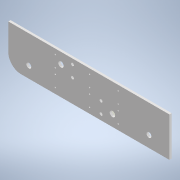
# Autodesk Inventor part: new sidewall inside
Saved by Autodesk Inventor 2020 (Build 240168000, 168)
## iProperties
Created: 2020-02-26
Part Number: new sidewall inside
Material: Generic
Document SubType Name: Modeling
Designer: jackm
Density: 1 g/cm^3
Appearance: Default
Author: jackm
Autodesk Inventor part; units mm, degrees
ref_plane "YZ Plane" through (0, 0, 0) normal (1, 0, 0) x (0, 1, 0)
ref_plane "XZ Plane" through (0, 0, 0) normal (0, 1, 0) x (-1, 0, 0)
ref_plane "XY Plane" through (0, 0, 0) normal (0, 0, 1) x (1, 0, 0)
ref_plane "Work Plane1" through (0, 0, 0) normal (0, 0, 1) x (1, 0, 0)
sketch "Sketch1" plane through (0, 0, 0) normal (0, 0, 1) x (1, 0, 0)
  circle A0 centre (104, 56) radius 1.778 construction
  circle A1 centre (104, 88) radius 1.778 construction
  circle A2 centre (184, 88) radius 1.778 construction
  line L0 (327.4055, 102.35) -> (327.4055, -7.6771) construction
  line L1 (-123.4445, 102.35) -> (327.4055, 102.35) construction
  line L2 (-123.4445, 27.6143) -> (-123.4445, 102.35) construction
  arc A3 (-123.4445, 27.6143) -> (-88.1531, -7.6771) centre (-88.1531, 27.6143) ccw construction
  line L3 (327.4055, -7.6771) -> (-88.1531, -7.6771) construction
  circle A4 centre (270.0149, 24.0729) radius 6.8857 construction
  circle A5 centre (-66.0538, 24.0729) radius 6.8834 construction
  circle A6 centre (168.0148, 24) radius 6.8834 construction
  circle A7 centre (23.9852, 72) radius 6.8834 construction
  line L4 (-123.4445, 102.35) -> (327.4055, 102.35)
  line L5 (327.4055, 102.35) -> (327.4055, -7.6771)
  line L6 (327.4055, -7.6771) -> (-88.1531, -7.6771)
  line L7 (-123.4445, 27.6143) -> (-123.4445, 102.35)
  arc A8 (-123.4445, 27.6143) -> (-88.1531, -7.6771) centre (-88.1531, 27.6143) ccw
  circle A9 centre (-66.0538, 24.0729) radius 6.8834
  circle A10 centre (270.0149, 24.0729) radius 6.8857
  circle A11 centre (23.9852, 72) radius 7.62
  circle A12 centre (168.0148, 24) radius 7.62
  circle A13 centre (56, 56) radius 3.5 construction
  circle A14 centre (136, 40) radius 3.5 construction
  circle A15 centre (136, 8) radius 3.5 construction
  circle A16 centre (56, 88) radius 3.5 construction
  circle A17 centre (56, 88) radius 4.064
  circle A18 centre (56, 56) radius 4.064
  circle A19 centre (136, 40) radius 4.064
  circle A20 centre (136, 8) radius 4.064
  line L8 (192, 0) -> (192, 48) construction
  line L9 (0, 48) -> (192, 48) construction
  line L10 (0, 0) -> (0, 48) construction
  line L11 (0, 0) -> (192, 0) construction
  circle A21 centre (168, 24) radius 7 construction
  circle A22 centre (144, 24) radius 7 construction
  arc A23 (160.9289, 33.8995) -> (158.1005, 31.0711) centre (159.5147, 32.4853) ccw construction
  line L12 (161.4142, 33.4142) -> (160.9289, 33.8995) construction
  arc A24 (158.5858, 30.5858) -> (161.4142, 33.4142) centre (160, 32) ccw construction
  line L13 (158.1005, 31.0711) -> (158.5858, 30.5858) construction
  line L14 (155.3137, 22) -> (156.6863, 22) construction
  arc A25 (155.3137, 26) -> (155.3137, 22) centre (155.3137, 24) ccw construction
  line L15 (156.6863, 26) -> (155.3137, 26) construction
  arc A26 (156.6863, 22) -> (156.6863, 26) centre (156.6863, 24) ccw construction
  arc A27 (158.1005, 16.9289) -> (160.9289, 14.1005) centre (159.5147, 15.5147) ccw construction
  line L16 (158.5858, 17.4142) -> (158.1005, 16.9289) construction
  arc A28 (161.4142, 14.5858) -> (158.5858, 17.4142) centre (160, 16) ccw construction
  line L17 (160.9289, 14.1005) -> (161.4142, 14.5858) construction
  arc A29 (177.8995, 31.0711) -> (175.0711, 33.8995) centre (176.4853, 32.4853) ccw construction
  line L18 (177.4142, 30.5858) -> (177.8995, 31.0711) construction
  arc A30 (174.5858, 33.4142) -> (177.4142, 30.5858) centre (176, 32) ccw construction
  line L19 (175.0711, 33.8995) -> (174.5858, 33.4142) construction
  line L20 (180.6863, 26) -> (179.3137, 26) construction
  arc A31 (180.6863, 22) -> (180.6863, 26) centre (180.6863, 24) ccw construction
  line L21 (179.3137, 22) -> (180.6863, 22) construction
  arc A32 (179.3137, 26) -> (179.3137, 22) centre (179.3137, 24) ccw construction
  line L22 (170, 35.3137) -> (170, 40) construction
  arc A33 (166, 35.3137) -> (170, 35.3137) centre (168, 35.3137) ccw construction
  line L23 (166, 40) -> (166, 35.3137) construction
  arc A34 (170, 40) -> (166, 40) centre (168, 40) ccw construction
  circle A35 centre (160, 40) radius 2 construction
  circle A36 centre (152, 40) radius 2 construction
  line L24 (146, 35.3137) -> (146, 40) construction
  arc A37 (142, 35.3137) -> (146, 35.3137) centre (144, 35.3137) ccw construction
  line L25 (142, 40) -> (142, 35.3137) construction
  arc A38 (146, 40) -> (142, 40) centre (144, 40) ccw construction
  circle A39 centre (136, 40) radius 2 construction
  circle A40 centre (128, 40) radius 2 construction
  line L26 (122, 35.3137) -> (122, 40) construction
  arc A41 (118, 35.3137) -> (122, 35.3137) centre (120, 35.3137) ccw construction
  line L27 (118, 40) -> (118, 35.3137) construction
  arc A42 (122, 40) -> (118, 40) centre (120, 40) ccw construction
  circle A43 centre (112, 40) radius 2 construction
  circle A44 centre (104, 40) radius 2 construction
  line L28 (98, 35.3137) -> (98, 40) construction
  arc A45 (94, 35.3137) -> (98, 35.3137) centre (96, 35.3137) ccw construction
  line L29 (94, 40) -> (94, 35.3137) construction
  arc A46 (98, 40) -> (94, 40) centre (96, 40) ccw construction
  circle A47 centre (88, 40) radius 2 construction
  circle A48 centre (80, 40) radius 2 construction
  line L30 (74, 35.3137) -> (74, 40) construction
  arc A49 (70, 35.3137) -> (74, 35.3137) centre (72, 35.3137) ccw construction
  line L31 (70, 40) -> (70, 35.3137) construction
  arc A50 (74, 40) -> (70, 40) centre (72, 40) ccw construction
  circle A51 centre (64, 40) radius 2 construction
  circle A52 centre (56, 40) radius 2 construction
  line L32 (50, 35.3137) -> (50, 40) construction
  arc A53 (46, 35.3137) -> (50, 35.3137) centre (48, 35.3137) ccw construction
  line L33 (46, 40) -> (46, 35.3137) construction
  arc A54 (50, 40) -> (46, 40) centre (48, 40) ccw construction
  circle A55 centre (40, 40) radius 2 construction
  circle A56 centre (32, 40) radius 2 construction
  line L34 (26, 35.3137) -> (26, 40) construction
  arc A57 (22, 35.3137) -> (26, 35.3137) centre (24, 35.3137) ccw construction
  line L35 (22, 40) -> (22, 35.3137) construction
  arc A58 (26, 40) -> (22, 40) centre (24, 40) ccw construction
  circle A59 centre (16, 40) radius 2 construction
  circle A60 centre (8, 40) radius 2 construction
  line L36 (166, 12.6863) -> (166, 8) construction
  arc A61 (170, 12.6863) -> (166, 12.6863) centre (168, 12.6863) ccw construction
  line L37 (170, 8) -> (170, 12.6863) construction
  arc A62 (166, 8) -> (170, 8) centre (168, 8) ccw construction
  circle A63 centre (160, 8) radius 2 construction
  circle A64 centre (152, 8) radius 2 construction
  line L38 (142, 12.6863) -> (142, 8) construction
  arc A65 (146, 12.6863) -> (142, 12.6863) centre (144, 12.6863) ccw construction
  line L39 (146, 8) -> (146, 12.6863) construction
  arc A66 (142, 8) -> (146, 8) centre (144, 8) ccw construction
  circle A67 centre (136, 8) radius 2 construction
  circle A68 centre (128, 8) radius 2 construction
  line L40 (118, 12.6863) -> (118, 8) construction
  arc A69 (122, 12.6863) -> (118, 12.6863) centre (120, 12.6863) ccw construction
  line L41 (122, 8) -> (122, 12.6863) construction
  arc A70 (118, 8) -> (122, 8) centre (120, 8) ccw construction
  circle A71 centre (112, 8) radius 2 construction
  circle A72 centre (104, 8) radius 2 construction
  line L42 (94, 12.6863) -> (94, 8) construction
  arc A73 (98, 12.6863) -> (94, 12.6863) centre (96, 12.6863) ccw construction
  line L43 (98, 8) -> (98, 12.6863) construction
  arc A74 (94, 8) -> (98, 8) centre (96, 8) ccw construction
  circle A75 centre (88, 8) radius 2 construction
  circle A76 centre (80, 8) radius 2 construction
  line L44 (70, 12.6863) -> (70, 8) construction
  arc A77 (74, 12.6863) -> (70, 12.6863) centre (72, 12.6863) ccw construction
  line L45 (74, 8) -> (74, 12.6863) construction
  arc A78 (70, 8) -> (74, 8) centre (72, 8) ccw construction
  circle A79 centre (64, 8) radius 2 construction
  circle A80 centre (56, 8) radius 2 construction
  line L46 (46, 12.6863) -> (46, 8) construction
  arc A81 (50, 12.6863) -> (46, 12.6863) centre (48, 12.6863) ccw construction
  line L47 (50, 8) -> (50, 12.6863) construction
  arc A82 (46, 8) -> (50, 8) centre (48, 8) ccw construction
  circle A83 centre (40, 8) radius 2 construction
  circle A84 centre (32, 8) radius 2 construction
  line L48 (22, 12.6863) -> (22, 8) construction
  arc A85 (26, 12.6863) -> (22, 12.6863) centre (24, 12.6863) ccw construction
  line L49 (26, 8) -> (26, 12.6863) construction
  arc A86 (22, 8) -> (26, 8) centre (24, 8) ccw construction
  circle A87 centre (16, 8) radius 2 construction
  circle A88 centre (8, 8) radius 2 construction
  arc A89 (9.8995, 31.0711) -> (7.0711, 33.8995) centre (8.4853, 32.4853) ccw construction
  line L50 (9.4142, 30.5858) -> (9.8995, 31.0711) construction
  arc A90 (6.5858, 33.4142) -> (9.4142, 30.5858) centre (8, 32) ccw construction
  line L51 (7.0711, 33.8995) -> (6.5858, 33.4142) construction
  arc A91 (7.0711, 14.1005) -> (9.8995, 16.9289) centre (8.4853, 15.5147) ccw construction
  line L52 (6.5858, 14.5858) -> (7.0711, 14.1005) construction
  arc A92 (9.4142, 17.4142) -> (6.5858, 14.5858) centre (8, 16) ccw construction
  line L53 (9.8995, 16.9289) -> (9.4142, 17.4142) construction
  arc A93 (184.9289, 33.8995) -> (182.1005, 31.0711) centre (183.5147, 32.4853) ccw construction
  line L54 (185.4142, 33.4142) -> (184.9289, 33.8995) construction
  arc A94 (182.5858, 30.5858) -> (185.4142, 33.4142) centre (184, 32) ccw construction
  line L55 (182.1005, 31.0711) -> (182.5858, 30.5858) construction
  arc A95 (182.1005, 16.9289) -> (184.9289, 14.1005) centre (183.5147, 15.5147) ccw construction
  line L56 (182.5858, 17.4142) -> (182.1005, 16.9289) construction
  arc A96 (185.4142, 14.5858) -> (182.5858, 17.4142) centre (184, 16) ccw construction
  line L57 (184.9289, 14.1005) -> (185.4142, 14.5858) construction
  circle A97 centre (176, 8) radius 2 construction
  circle A98 centre (176, 40) radius 2 construction
  circle A99 centre (184, 40) radius 2 construction
  circle A100 centre (184, 8) radius 2 construction
  arc A101 (33.8995, 31.0711) -> (31.0711, 33.8995) centre (32.4853, 32.4853) ccw construction
  line L58 (33.4142, 30.5858) -> (33.8995, 31.0711) construction
  arc A102 (30.5858, 33.4142) -> (33.4142, 30.5858) centre (32, 32) ccw construction
  line L59 (31.0711, 33.8995) -> (30.5858, 33.4142) construction
  arc A103 (57.8995, 31.0711) -> (55.0711, 33.8995) centre (56.4853, 32.4853) ccw construction
  line L60 (57.4142, 30.5858) -> (57.8995, 31.0711) construction
  arc A104 (54.5858, 33.4142) -> (57.4142, 30.5858) centre (56, 32) ccw construction
  line L61 (55.0711, 33.8995) -> (54.5858, 33.4142) construction
  arc A105 (81.8995, 31.0711) -> (79.0711, 33.8995) centre (80.4853, 32.4853) ccw construction
  line L62 (81.4142, 30.5858) -> (81.8995, 31.0711) construction
  arc A106 (78.5858, 33.4142) -> (81.4142, 30.5858) centre (80, 32) ccw construction
  line L63 (79.0711, 33.8995) -> (78.5858, 33.4142) construction
  arc A107 (105.8995, 31.0711) -> (103.0711, 33.8995) centre (104.4853, 32.4853) ccw construction
  line L64 (105.4142, 30.5858) -> (105.8995, 31.0711) construction
  arc A108 (102.5858, 33.4142) -> (105.4142, 30.5858) centre (104, 32) ccw construction
  line L65 (103.0711, 33.8995) -> (102.5858, 33.4142) construction
  arc A109 (129.8995, 31.0711) -> (127.0711, 33.8995) centre (128.4853, 32.4853) ccw construction
  line L66 (129.4142, 30.5858) -> (129.8995, 31.0711) construction
  arc A110 (126.5858, 33.4142) -> (129.4142, 30.5858) centre (128, 32) ccw construction
  line L67 (127.0711, 33.8995) -> (126.5858, 33.4142) construction
  arc A111 (153.8995, 31.0711) -> (151.0711, 33.8995) centre (152.4853, 32.4853) ccw construction
  line L68 (153.4142, 30.5858) -> (153.8995, 31.0711) construction
  arc A112 (150.5858, 33.4142) -> (153.4142, 30.5858) centre (152, 32) ccw construction
  line L69 (151.0711, 33.8995) -> (150.5858, 33.4142) construction
  arc A113 (14.1005, 16.9289) -> (16.9289, 14.1005) centre (15.5147, 15.5147) ccw construction
  line L70 (14.5858, 17.4142) -> (14.1005, 16.9289) construction
  arc A114 (17.4142, 14.5858) -> (14.5858, 17.4142) centre (16, 16) ccw construction
  line L71 (16.9289, 14.1005) -> (17.4142, 14.5858) construction
  arc A115 (38.1005, 16.9289) -> (40.9289, 14.1005) centre (39.5147, 15.5147) ccw construction
  line L72 (38.5858, 17.4142) -> (38.1005, 16.9289) construction
  arc A116 (41.4142, 14.5858) -> (38.5858, 17.4142) centre (40, 16) ccw construction
  line L73 (40.9289, 14.1005) -> (41.4142, 14.5858) construction
  arc A117 (62.1005, 16.9289) -> (64.9289, 14.1005) centre (63.5147, 15.5147) ccw construction
  line L74 (62.5858, 17.4142) -> (62.1005, 16.9289) construction
  arc A118 (65.4142, 14.5858) -> (62.5858, 17.4142) centre (64, 16) ccw construction
  line L75 (64.9289, 14.1005) -> (65.4142, 14.5858) construction
  arc A119 (86.1005, 16.9289) -> (88.9289, 14.1005) centre (87.5147, 15.5147) ccw construction
  line L76 (86.5858, 17.4142) -> (86.1005, 16.9289) construction
  arc A120 (89.4142, 14.5858) -> (86.5858, 17.4142) centre (88, 16) ccw construction
  line L77 (88.9289, 14.1005) -> (89.4142, 14.5858) construction
  arc A121 (110.1005, 16.9289) -> (112.9289, 14.1005) centre (111.5147, 15.5147) ccw construction
  line L78 (110.5858, 17.4142) -> (110.1005, 16.9289) construction
  arc A122 (113.4142, 14.5858) -> (110.5858, 17.4142) centre (112, 16) ccw construction
  line L79 (112.9289, 14.1005) -> (113.4142, 14.5858) construction
  arc A123 (134.1005, 16.9289) -> (136.9289, 14.1005) centre (135.5147, 15.5147) ccw construction
  line L80 (134.5858, 17.4142) -> (134.1005, 16.9289) construction
  arc A124 (137.4142, 14.5858) -> (134.5858, 17.4142) centre (136, 16) ccw construction
  line L81 (136.9289, 14.1005) -> (137.4142, 14.5858) construction
  arc A125 (11.3137, 26) -> (11.3137, 22) centre (11.3137, 24) ccw construction
  line L82 (12.6863, 26) -> (11.3137, 26) construction
  arc A126 (12.6863, 22) -> (12.6863, 26) centre (12.6863, 24) ccw construction
  line L83 (11.3137, 22) -> (12.6863, 22) construction
  line L84 (35.3137, 22) -> (36.6863, 22) construction
  arc A127 (35.3137, 26) -> (35.3137, 22) centre (35.3137, 24) ccw construction
  line L85 (36.6863, 26) -> (35.3137, 26) construction
  arc A128 (36.6863, 22) -> (36.6863, 26) centre (36.6863, 24) ccw construction
  line L86 (59.3137, 22) -> (60.6863, 22) construction
  arc A129 (59.3137, 26) -> (59.3137, 22) centre (59.3137, 24) ccw construction
  line L87 (60.6863, 26) -> (59.3137, 26) construction
  arc A130 (60.6863, 22) -> (60.6863, 26) centre (60.6863, 24) ccw construction
  line L88 (83.3137, 22) -> (84.6863, 22) construction
  arc A131 (83.3137, 26) -> (83.3137, 22) centre (83.3137, 24) ccw construction
  line L89 (84.6863, 26) -> (83.3137, 26) construction
  arc A132 (84.6863, 22) -> (84.6863, 26) centre (84.6863, 24) ccw construction
  line L90 (107.3137, 22) -> (108.6863, 22) construction
  arc A133 (107.3137, 26) -> (107.3137, 22) centre (107.3137, 24) ccw construction
  line L91 (108.6863, 26) -> (107.3137, 26) construction
  arc A134 (108.6863, 22) -> (108.6863, 26) centre (108.6863, 24) ccw construction
  line L92 (131.3137, 22) -> (132.6863, 22) construction
  arc A135 (131.3137, 26) -> (131.3137, 22) centre (131.3137, 24) ccw construction
  line L93 (132.6863, 26) -> (131.3137, 26) construction
  arc A136 (132.6863, 22) -> (132.6863, 26) centre (132.6863, 24) ccw construction
  arc A137 (16.9289, 33.8995) -> (14.1005, 31.0711) centre (15.5147, 32.4853) ccw construction
  line L94 (17.4142, 33.4142) -> (16.9289, 33.8995) construction
  arc A138 (14.5858, 30.5858) -> (17.4142, 33.4142) centre (16, 32) ccw construction
  line L95 (14.1005, 31.0711) -> (14.5858, 30.5858) construction
  arc A139 (40.9289, 33.8995) -> (38.1005, 31.0711) centre (39.5147, 32.4853) ccw construction
  line L96 (41.4142, 33.4142) -> (40.9289, 33.8995) construction
  arc A140 (38.5858, 30.5858) -> (41.4142, 33.4142) centre (40, 32) ccw construction
  line L97 (38.1005, 31.0711) -> (38.5858, 30.5858) construction
  arc A141 (64.9289, 33.8995) -> (62.1005, 31.0711) centre (63.5147, 32.4853) ccw construction
  line L98 (65.4142, 33.4142) -> (64.9289, 33.8995) construction
  arc A142 (62.5858, 30.5858) -> (65.4142, 33.4142) centre (64, 32) ccw construction
  line L99 (62.1005, 31.0711) -> (62.5858, 30.5858) construction
  arc A143 (88.9289, 33.8995) -> (86.1005, 31.0711) centre (87.5147, 32.4853) ccw construction
  line L100 (89.4142, 33.4142) -> (88.9289, 33.8995) construction
  arc A144 (86.5858, 30.5858) -> (89.4142, 33.4142) centre (88, 32) ccw construction
  line L101 (86.1005, 31.0711) -> (86.5858, 30.5858) construction
  arc A145 (112.9289, 33.8995) -> (110.1005, 31.0711) centre (111.5147, 32.4853) ccw construction
  line L102 (113.4142, 33.4142) -> (112.9289, 33.8995) construction
  arc A146 (110.5858, 30.5858) -> (113.4142, 33.4142) centre (112, 32) ccw construction
  line L103 (110.1005, 31.0711) -> (110.5858, 30.5858) construction
  arc A147 (136.9289, 33.8995) -> (134.1005, 31.0711) centre (135.5147, 32.4853) ccw construction
  line L104 (137.4142, 33.4142) -> (136.9289, 33.8995) construction
  arc A148 (134.5858, 30.5858) -> (137.4142, 33.4142) centre (136, 32) ccw construction
  line L105 (134.1005, 31.0711) -> (134.5858, 30.5858) construction
  arc A149 (31.0711, 14.1005) -> (33.8995, 16.9289) centre (32.4853, 15.5147) ccw construction
  line L106 (30.5858, 14.5858) -> (31.0711, 14.1005) construction
  arc A150 (33.4142, 17.4142) -> (30.5858, 14.5858) centre (32, 16) ccw construction
  line L107 (33.8995, 16.9289) -> (33.4142, 17.4142) construction
  arc A151 (55.0711, 14.1005) -> (57.8995, 16.9289) centre (56.4853, 15.5147) ccw construction
  line L108 (54.5858, 14.5858) -> (55.0711, 14.1005) construction
  arc A152 (57.4142, 17.4142) -> (54.5858, 14.5858) centre (56, 16) ccw construction
  line L109 (57.8995, 16.9289) -> (57.4142, 17.4142) construction
  arc A153 (79.0711, 14.1005) -> (81.8995, 16.9289) centre (80.4853, 15.5147) ccw construction
  line L110 (78.5858, 14.5858) -> (79.0711, 14.1005) construction
  arc A154 (81.4142, 17.4142) -> (78.5858, 14.5858) centre (80, 16) ccw construction
  line L111 (81.8995, 16.9289) -> (81.4142, 17.4142) construction
  arc A155 (103.0711, 14.1005) -> (105.8995, 16.9289) centre (104.4853, 15.5147) ccw construction
  line L112 (102.5858, 14.5858) -> (103.0711, 14.1005) construction
  arc A156 (105.4142, 17.4142) -> (102.5858, 14.5858) centre (104, 16) ccw construction
  line L113 (105.8995, 16.9289) -> (105.4142, 17.4142) construction
  arc A157 (127.0711, 14.1005) -> (129.8995, 16.9289) centre (128.4853, 15.5147) ccw construction
  line L114 (126.5858, 14.5858) -> (127.0711, 14.1005) construction
  arc A158 (129.4142, 17.4142) -> (126.5858, 14.5858) centre (128, 16) ccw construction
  line L115 (129.8995, 16.9289) -> (129.4142, 17.4142) construction
  arc A159 (151.0711, 14.1005) -> (153.8995, 16.9289) centre (152.4853, 15.5147) ccw construction
  line L116 (150.5858, 14.5858) -> (151.0711, 14.1005) construction
  arc A160 (153.4142, 17.4142) -> (150.5858, 14.5858) centre (152, 16) ccw construction
  line L117 (153.8995, 16.9289) -> (153.4142, 17.4142) construction
  arc A161 (175.0711, 14.1005) -> (177.8995, 16.9289) centre (176.4853, 15.5147) ccw construction
  line L118 (174.5858, 14.5858) -> (175.0711, 14.1005) construction
  arc A162 (177.4142, 17.4142) -> (174.5858, 14.5858) centre (176, 16) ccw construction
  line L119 (177.8995, 16.9289) -> (177.4142, 17.4142) construction
  circle A163 centre (24, 24) radius 7 construction
  circle A164 centre (48, 24) radius 7 construction
  circle A165 centre (72, 24) radius 7 construction
  circle A166 centre (96, 24) radius 7 construction
  circle A167 centre (120, 24) radius 7 construction
  line L120 (0, 96) -> (0, 48) construction
  line L121 (192, 48) -> (0, 48) construction
  line L122 (192, 96) -> (192, 48) construction
  line L123 (192, 96) -> (0, 96) construction
  circle A168 centre (24, 72) radius 7 construction
  circle A169 centre (48, 72) radius 7 construction
  arc A170 (31.0711, 62.1005) -> (33.8995, 64.9289) centre (32.4853, 63.5147) ccw construction
  line L124 (30.5858, 62.5858) -> (31.0711, 62.1005) construction
  arc A171 (33.4142, 65.4142) -> (30.5858, 62.5858) centre (32, 64) ccw construction
  line L125 (33.8995, 64.9289) -> (33.4142, 65.4142) construction
  line L126 (36.6863, 74) -> (35.3137, 74) construction
  arc A172 (36.6863, 70) -> (36.6863, 74) centre (36.6863, 72) ccw construction
  line L127 (35.3137, 70) -> (36.6863, 70) construction
  arc A173 (35.3137, 74) -> (35.3137, 70) centre (35.3137, 72) ccw construction
  arc A174 (33.8995, 79.0711) -> (31.0711, 81.8995) centre (32.4853, 80.4853) ccw construction
  line L128 (33.4142, 78.5858) -> (33.8995, 79.0711) construction
  arc A175 (30.5858, 81.4142) -> (33.4142, 78.5858) centre (32, 80) ccw construction
  line L129 (31.0711, 81.8995) -> (30.5858, 81.4142) construction
  arc A176 (14.1005, 64.9289) -> (16.9289, 62.1005) centre (15.5147, 63.5147) ccw construction
  line L130 (14.5858, 65.4142) -> (14.1005, 64.9289) construction
  arc A177 (17.4142, 62.5858) -> (14.5858, 65.4142) centre (16, 64) ccw construction
  line L131 (16.9289, 62.1005) -> (17.4142, 62.5858) construction
  line L132 (11.3137, 70) -> (12.6863, 70) construction
  arc A178 (11.3137, 74) -> (11.3137, 70) centre (11.3137, 72) ccw construction
  line L133 (12.6863, 74) -> (11.3137, 74) construction
  arc A179 (12.6863, 70) -> (12.6863, 74) centre (12.6863, 72) ccw construction
  line L134 (22, 60.6863) -> (22, 56) construction
  arc A180 (26, 60.6863) -> (22, 60.6863) centre (24, 60.6863) ccw construction
  line L135 (26, 56) -> (26, 60.6863) construction
  arc A181 (22, 56) -> (26, 56) centre (24, 56) ccw construction
  circle A182 centre (32, 56) radius 2 construction
  circle A183 centre (40, 56) radius 2 construction
  line L136 (46, 60.6863) -> (46, 56) construction
  arc A184 (50, 60.6863) -> (46, 60.6863) centre (48, 60.6863) ccw construction
  line L137 (50, 56) -> (50, 60.6863) construction
  arc A185 (46, 56) -> (50, 56) centre (48, 56) ccw construction
  circle A186 centre (56, 56) radius 2 construction
  circle A187 centre (64, 56) radius 2 construction
  line L138 (70, 60.6863) -> (70, 56) construction
  arc A188 (74, 60.6863) -> (70, 60.6863) centre (72, 60.6863) ccw construction
  line L139 (74, 56) -> (74, 60.6863) construction
  arc A189 (70, 56) -> (74, 56) centre (72, 56) ccw construction
  circle A190 centre (80, 56) radius 2 construction
  circle A191 centre (88, 56) radius 2 construction
  line L140 (94, 60.6863) -> (94, 56) construction
  arc A192 (98, 60.6863) -> (94, 60.6863) centre (96, 60.6863) ccw construction
  line L141 (98, 56) -> (98, 60.6863) construction
  arc A193 (94, 56) -> (98, 56) centre (96, 56) ccw construction
  circle A194 centre (104, 56) radius 2 construction
  circle A195 centre (112, 56) radius 2 construction
  line L142 (118, 60.6863) -> (118, 56) construction
  arc A196 (122, 60.6863) -> (118, 60.6863) centre (120, 60.6863) ccw construction
  line L143 (122, 56) -> (122, 60.6863) construction
  arc A197 (118, 56) -> (122, 56) centre (120, 56) ccw construction
  circle A198 centre (128, 56) radius 2 construction
  circle A199 centre (136, 56) radius 2 construction
  line L144 (142, 60.6863) -> (142, 56) construction
  arc A200 (146, 60.6863) -> (142, 60.6863) centre (144, 60.6863) ccw construction
  line L145 (146, 56) -> (146, 60.6863) construction
  arc A201 (142, 56) -> (146, 56) centre (144, 56) ccw construction
  circle A202 centre (152, 56) radius 2 construction
  circle A203 centre (160, 56) radius 2 construction
  line L146 (166, 60.6863) -> (166, 56) construction
  arc A204 (170, 60.6863) -> (166, 60.6863) centre (168, 60.6863) ccw construction
  line L147 (170, 56) -> (170, 60.6863) construction
  arc A205 (166, 56) -> (170, 56) centre (168, 56) ccw construction
  circle A206 centre (176, 56) radius 2 construction
  circle A207 centre (184, 56) radius 2 construction
  line L148 (26, 83.3137) -> (26, 88) construction
  arc A208 (22, 83.3137) -> (26, 83.3137) centre (24, 83.3137) ccw construction
  line L149 (22, 88) -> (22, 83.3137) construction
  arc A209 (26, 88) -> (22, 88) centre (24, 88) ccw construction
  circle A210 centre (32, 88) radius 2 construction
  circle A211 centre (40, 88) radius 2 construction
  line L150 (50, 83.3137) -> (50, 88) construction
  arc A212 (46, 83.3137) -> (50, 83.3137) centre (48, 83.3137) ccw construction
  line L151 (46, 88) -> (46, 83.3137) construction
  arc A213 (50, 88) -> (46, 88) centre (48, 88) ccw construction
  circle A214 centre (56, 88) radius 2 construction
  circle A215 centre (64, 88) radius 2 construction
  line L152 (74, 83.3137) -> (74, 88) construction
  arc A216 (70, 83.3137) -> (74, 83.3137) centre (72, 83.3137) ccw construction
  line L153 (70, 88) -> (70, 83.3137) construction
  arc A217 (74, 88) -> (70, 88) centre (72, 88) ccw construction
  circle A218 centre (80, 88) radius 2 construction
  circle A219 centre (88, 88) radius 2 construction
  line L154 (98, 83.3137) -> (98, 88) construction
  arc A220 (94, 83.3137) -> (98, 83.3137) centre (96, 83.3137) ccw construction
  line L155 (94, 88) -> (94, 83.3137) construction
  arc A221 (98, 88) -> (94, 88) centre (96, 88) ccw construction
  circle A222 centre (104, 88) radius 2 construction
  circle A223 centre (112, 88) radius 2 construction
  line L156 (122, 83.3137) -> (122, 88) construction
  arc A224 (118, 83.3137) -> (122, 83.3137) centre (120, 83.3137) ccw construction
  line L157 (118, 88) -> (118, 83.3137) construction
  arc A225 (122, 88) -> (118, 88) centre (120, 88) ccw construction
  circle A226 centre (128, 88) radius 2 construction
  circle A227 centre (136, 88) radius 2 construction
  line L158 (146, 83.3137) -> (146, 88) construction
  arc A228 (142, 83.3137) -> (146, 83.3137) centre (144, 83.3137) ccw construction
  line L159 (142, 88) -> (142, 83.3137) construction
  arc A229 (146, 88) -> (142, 88) centre (144, 88) ccw construction
  circle A230 centre (152, 88) radius 2 construction
  circle A231 centre (160, 88) radius 2 construction
  line L160 (170, 83.3137) -> (170, 88) construction
  arc A232 (166, 83.3137) -> (170, 83.3137) centre (168, 83.3137) ccw construction
  line L161 (166, 88) -> (166, 83.3137) construction
  arc A233 (170, 88) -> (166, 88) centre (168, 88) ccw construction
  circle A234 centre (176, 88) radius 2 construction
  circle A235 centre (184, 88) radius 2 construction
  arc A236 (182.1005, 64.9289) -> (184.9289, 62.1005) centre (183.5147, 63.5147) ccw construction
  line L162 (182.5858, 65.4142) -> (182.1005, 64.9289) construction
  arc A237 (185.4142, 62.5858) -> (182.5858, 65.4142) centre (184, 64) ccw construction
  line L163 (184.9289, 62.1005) -> (185.4142, 62.5858) construction
  arc A238 (184.9289, 81.8995) -> (182.1005, 79.0711) centre (183.5147, 80.4853) ccw construction
  line L164 (185.4142, 81.4142) -> (184.9289, 81.8995) construction
  arc A239 (182.5858, 78.5858) -> (185.4142, 81.4142) centre (184, 80) ccw construction
  line L165 (182.1005, 79.0711) -> (182.5858, 78.5858) construction
  arc A240 (7.0711, 62.1005) -> (9.8995, 64.9289) centre (8.4853, 63.5147) ccw construction
  line L166 (6.5858, 62.5858) -> (7.0711, 62.1005) construction
  arc A241 (9.4142, 65.4142) -> (6.5858, 62.5858) centre (8, 64) ccw construction
  line L167 (9.8995, 64.9289) -> (9.4142, 65.4142) construction
  arc A242 (9.8995, 79.0711) -> (7.0711, 81.8995) centre (8.4853, 80.4853) ccw construction
  line L168 (9.4142, 78.5858) -> (9.8995, 79.0711) construction
  arc A243 (6.5858, 81.4142) -> (9.4142, 78.5858) centre (8, 80) ccw construction
  line L169 (7.0711, 81.8995) -> (6.5858, 81.4142) construction
  circle A244 centre (16, 88) radius 2 construction
  circle A245 centre (16, 56) radius 2 construction
  circle A246 centre (8, 56) radius 2 construction
  circle A247 centre (8, 88) radius 2 construction
  arc A248 (158.1005, 64.9289) -> (160.9289, 62.1005) centre (159.5147, 63.5147) ccw construction
  line L170 (158.5858, 65.4142) -> (158.1005, 64.9289) construction
  arc A249 (161.4142, 62.5858) -> (158.5858, 65.4142) centre (160, 64) ccw construction
  line L171 (160.9289, 62.1005) -> (161.4142, 62.5858) construction
  arc A250 (134.1005, 64.9289) -> (136.9289, 62.1005) centre (135.5147, 63.5147) ccw construction
  line L172 (134.5858, 65.4142) -> (134.1005, 64.9289) construction
  arc A251 (137.4142, 62.5858) -> (134.5858, 65.4142) centre (136, 64) ccw construction
  line L173 (136.9289, 62.1005) -> (137.4142, 62.5858) construction
  arc A252 (110.1005, 64.9289) -> (112.9289, 62.1005) centre (111.5147, 63.5147) ccw construction
  line L174 (110.5858, 65.4142) -> (110.1005, 64.9289) construction
  arc A253 (113.4142, 62.5858) -> (110.5858, 65.4142) centre (112, 64) ccw construction
  line L175 (112.9289, 62.1005) -> (113.4142, 62.5858) construction
  arc A254 (86.1005, 64.9289) -> (88.9289, 62.1005) centre (87.5147, 63.5147) ccw construction
  line L176 (86.5858, 65.4142) -> (86.1005, 64.9289) construction
  arc A255 (89.4142, 62.5858) -> (86.5858, 65.4142) centre (88, 64) ccw construction
  line L177 (88.9289, 62.1005) -> (89.4142, 62.5858) construction
  arc A256 (62.1005, 64.9289) -> (64.9289, 62.1005) centre (63.5147, 63.5147) ccw construction
  line L178 (62.5858, 65.4142) -> (62.1005, 64.9289) construction
  arc A257 (65.4142, 62.5858) -> (62.5858, 65.4142) centre (64, 64) ccw construction
  line L179 (64.9289, 62.1005) -> (65.4142, 62.5858) construction
  arc A258 (38.1005, 64.9289) -> (40.9289, 62.1005) centre (39.5147, 63.5147) ccw construction
  line L180 (38.5858, 65.4142) -> (38.1005, 64.9289) construction
  arc A259 (41.4142, 62.5858) -> (38.5858, 65.4142) centre (40, 64) ccw construction
  line L181 (40.9289, 62.1005) -> (41.4142, 62.5858) construction
  arc A260 (177.8995, 79.0711) -> (175.0711, 81.8995) centre (176.4853, 80.4853) ccw construction
  line L182 (177.4142, 78.5858) -> (177.8995, 79.0711) construction
  arc A261 (174.5858, 81.4142) -> (177.4142, 78.5858) centre (176, 80) ccw construction
  line L183 (175.0711, 81.8995) -> (174.5858, 81.4142) construction
  arc A262 (153.8995, 79.0711) -> (151.0711, 81.8995) centre (152.4853, 80.4853) ccw construction
  line L184 (153.4142, 78.5858) -> (153.8995, 79.0711) construction
  arc A263 (150.5858, 81.4142) -> (153.4142, 78.5858) centre (152, 80) ccw construction
  line L185 (151.0711, 81.8995) -> (150.5858, 81.4142) construction
  arc A264 (129.8995, 79.0711) -> (127.0711, 81.8995) centre (128.4853, 80.4853) ccw construction
  line L186 (129.4142, 78.5858) -> (129.8995, 79.0711) construction
  arc A265 (126.5858, 81.4142) -> (129.4142, 78.5858) centre (128, 80) ccw construction
  line L187 (127.0711, 81.8995) -> (126.5858, 81.4142) construction
  arc A266 (105.8995, 79.0711) -> (103.0711, 81.8995) centre (104.4853, 80.4853) ccw construction
  line L188 (105.4142, 78.5858) -> (105.8995, 79.0711) construction
  arc A267 (102.5858, 81.4142) -> (105.4142, 78.5858) centre (104, 80) ccw construction
  line L189 (103.0711, 81.8995) -> (102.5858, 81.4142) construction
  arc A268 (81.8995, 79.0711) -> (79.0711, 81.8995) centre (80.4853, 80.4853) ccw construction
  line L190 (81.4142, 78.5858) -> (81.8995, 79.0711) construction
  arc A269 (78.5858, 81.4142) -> (81.4142, 78.5858) centre (80, 80) ccw construction
  line L191 (79.0711, 81.8995) -> (78.5858, 81.4142) construction
  arc A270 (57.8995, 79.0711) -> (55.0711, 81.8995) centre (56.4853, 80.4853) ccw construction
  line L192 (57.4142, 78.5858) -> (57.8995, 79.0711) construction
  arc A271 (54.5858, 81.4142) -> (57.4142, 78.5858) centre (56, 80) ccw construction
  line L193 (55.0711, 81.8995) -> (54.5858, 81.4142) construction
  arc A272 (180.6863, 70) -> (180.6863, 74) centre (180.6863, 72) ccw construction
  line L194 (179.3137, 70) -> (180.6863, 70) construction
  arc A273 (179.3137, 74) -> (179.3137, 70) centre (179.3137, 72) ccw construction
  line L195 (180.6863, 74) -> (179.3137, 74) construction
  line L196 (156.6863, 74) -> (155.3137, 74) construction
  arc A274 (156.6863, 70) -> (156.6863, 74) centre (156.6863, 72) ccw construction
  line L197 (155.3137, 70) -> (156.6863, 70) construction
  arc A275 (155.3137, 74) -> (155.3137, 70) centre (155.3137, 72) ccw construction
  line L198 (132.6863, 74) -> (131.3137, 74) construction
  arc A276 (132.6863, 70) -> (132.6863, 74) centre (132.6863, 72) ccw construction
  line L199 (131.3137, 70) -> (132.6863, 70) construction
  arc A277 (131.3137, 74) -> (131.3137, 70) centre (131.3137, 72) ccw construction
  line L200 (108.6863, 74) -> (107.3137, 74) construction
  arc A278 (108.6863, 70) -> (108.6863, 74) centre (108.6863, 72) ccw construction
  line L201 (107.3137, 70) -> (108.6863, 70) construction
  arc A279 (107.3137, 74) -> (107.3137, 70) centre (107.3137, 72) ccw construction
  line L202 (84.6863, 74) -> (83.3137, 74) construction
  arc A280 (84.6863, 70) -> (84.6863, 74) centre (84.6863, 72) ccw construction
  line L203 (83.3137, 70) -> (84.6863, 70) construction
  arc A281 (83.3137, 74) -> (83.3137, 70) centre (83.3137, 72) ccw construction
  line L204 (60.6863, 74) -> (59.3137, 74) construction
  arc A282 (60.6863, 70) -> (60.6863, 74) centre (60.6863, 72) ccw construction
  line L205 (59.3137, 70) -> (60.6863, 70) construction
  arc A283 (59.3137, 74) -> (59.3137, 70) centre (59.3137, 72) ccw construction
  arc A284 (175.0711, 62.1005) -> (177.8995, 64.9289) centre (176.4853, 63.5147) ccw construction
  line L206 (174.5858, 62.5858) -> (175.0711, 62.1005) construction
  arc A285 (177.4142, 65.4142) -> (174.5858, 62.5858) centre (176, 64) ccw construction
  line L207 (177.8995, 64.9289) -> (177.4142, 65.4142) construction
  arc A286 (151.0711, 62.1005) -> (153.8995, 64.9289) centre (152.4853, 63.5147) ccw construction
  line L208 (150.5858, 62.5858) -> (151.0711, 62.1005) construction
  arc A287 (153.4142, 65.4142) -> (150.5858, 62.5858) centre (152, 64) ccw construction
  line L209 (153.8995, 64.9289) -> (153.4142, 65.4142) construction
  arc A288 (127.0711, 62.1005) -> (129.8995, 64.9289) centre (128.4853, 63.5147) ccw construction
  line L210 (126.5858, 62.5858) -> (127.0711, 62.1005) construction
  arc A289 (129.4142, 65.4142) -> (126.5858, 62.5858) centre (128, 64) ccw construction
  line L211 (129.8995, 64.9289) -> (129.4142, 65.4142) construction
  arc A290 (103.0711, 62.1005) -> (105.8995, 64.9289) centre (104.4853, 63.5147) ccw construction
  line L212 (102.5858, 62.5858) -> (103.0711, 62.1005) construction
  arc A291 (105.4142, 65.4142) -> (102.5858, 62.5858) centre (104, 64) ccw construction
  line L213 (105.8995, 64.9289) -> (105.4142, 65.4142) construction
  arc A292 (79.0711, 62.1005) -> (81.8995, 64.9289) centre (80.4853, 63.5147) ccw construction
  line L214 (78.5858, 62.5858) -> (79.0711, 62.1005) construction
  arc A293 (81.4142, 65.4142) -> (78.5858, 62.5858) centre (80, 64) ccw construction
  line L215 (81.8995, 64.9289) -> (81.4142, 65.4142) construction
  arc A294 (55.0711, 62.1005) -> (57.8995, 64.9289) centre (56.4853, 63.5147) ccw construction
  line L216 (54.5858, 62.5858) -> (55.0711, 62.1005) construction
  arc A295 (57.4142, 65.4142) -> (54.5858, 62.5858) centre (56, 64) ccw construction
  line L217 (57.8995, 64.9289) -> (57.4142, 65.4142) construction
  arc A296 (160.9289, 81.8995) -> (158.1005, 79.0711) centre (159.5147, 80.4853) ccw construction
  line L218 (161.4142, 81.4142) -> (160.9289, 81.8995) construction
  arc A297 (158.5858, 78.5858) -> (161.4142, 81.4142) centre (160, 80) ccw construction
  line L219 (158.1005, 79.0711) -> (158.5858, 78.5858) construction
  arc A298 (136.9289, 81.8995) -> (134.1005, 79.0711) centre (135.5147, 80.4853) ccw construction
  line L220 (137.4142, 81.4142) -> (136.9289, 81.8995) construction
  arc A299 (134.5858, 78.5858) -> (137.4142, 81.4142) centre (136, 80) ccw construction
  line L221 (134.1005, 79.0711) -> (134.5858, 78.5858) construction
  arc A300 (112.9289, 81.8995) -> (110.1005, 79.0711) centre (111.5147, 80.4853) ccw construction
  line L222 (113.4142, 81.4142) -> (112.9289, 81.8995) construction
  arc A301 (110.5858, 78.5858) -> (113.4142, 81.4142) centre (112, 80) ccw construction
  line L223 (110.1005, 79.0711) -> (110.5858, 78.5858) construction
  arc A302 (88.9289, 81.8995) -> (86.1005, 79.0711) centre (87.5147, 80.4853) ccw construction
  line L224 (89.4142, 81.4142) -> (88.9289, 81.8995) construction
  arc A303 (86.5858, 78.5858) -> (89.4142, 81.4142) centre (88, 80) ccw construction
  line L225 (86.1005, 79.0711) -> (86.5858, 78.5858) construction
  arc A304 (64.9289, 81.8995) -> (62.1005, 79.0711) centre (63.5147, 80.4853) ccw construction
  line L226 (65.4142, 81.4142) -> (64.9289, 81.8995) construction
  arc A305 (62.5858, 78.5858) -> (65.4142, 81.4142) centre (64, 80) ccw construction
  line L227 (62.1005, 79.0711) -> (62.5858, 78.5858) construction
  arc A306 (40.9289, 81.8995) -> (38.1005, 79.0711) centre (39.5147, 80.4853) ccw construction
  line L228 (41.4142, 81.4142) -> (40.9289, 81.8995) construction
  arc A307 (38.5858, 78.5858) -> (41.4142, 81.4142) centre (40, 80) ccw construction
  line L229 (38.1005, 79.0711) -> (38.5858, 78.5858) construction
  arc A308 (16.9289, 81.8995) -> (14.1005, 79.0711) centre (15.5147, 80.4853) ccw construction
  line L230 (17.4142, 81.4142) -> (16.9289, 81.8995) construction
  arc A309 (14.5858, 78.5858) -> (17.4142, 81.4142) centre (16, 80) ccw construction
  line L231 (14.1005, 79.0711) -> (14.5858, 78.5858) construction
  circle A310 centre (168, 72) radius 7 construction
  circle A311 centre (144, 72) radius 7 construction
  circle A312 centre (120, 72) radius 7 construction
  circle A313 centre (96, 72) radius 7 construction
  circle A314 centre (72, 72) radius 7 construction
  circle A315 centre (8, 88) radius 1.778
  circle A316 centre (8, 56) radius 1.778
  circle A317 centre (8, 40) radius 1.778
  circle A318 centre (8, 8) radius 1.778
  circle A319 centre (184, 88) radius 1.778
  circle A320 centre (184, 56) radius 1.778
  circle A321 centre (184, 40) radius 1.778
  circle A322 centre (184, 8) radius 1.778
  circle A323 centre (104, 56) radius 1.778
  circle A324 centre (104, 88) radius 1.778
  circle A325 centre (104, 40) radius 1.778
  circle A326 centre (104, 8) radius 1.778
extrude "Extrusion1" add sketch "Sketch1" along normal blind 6.35
body "Solid1"
